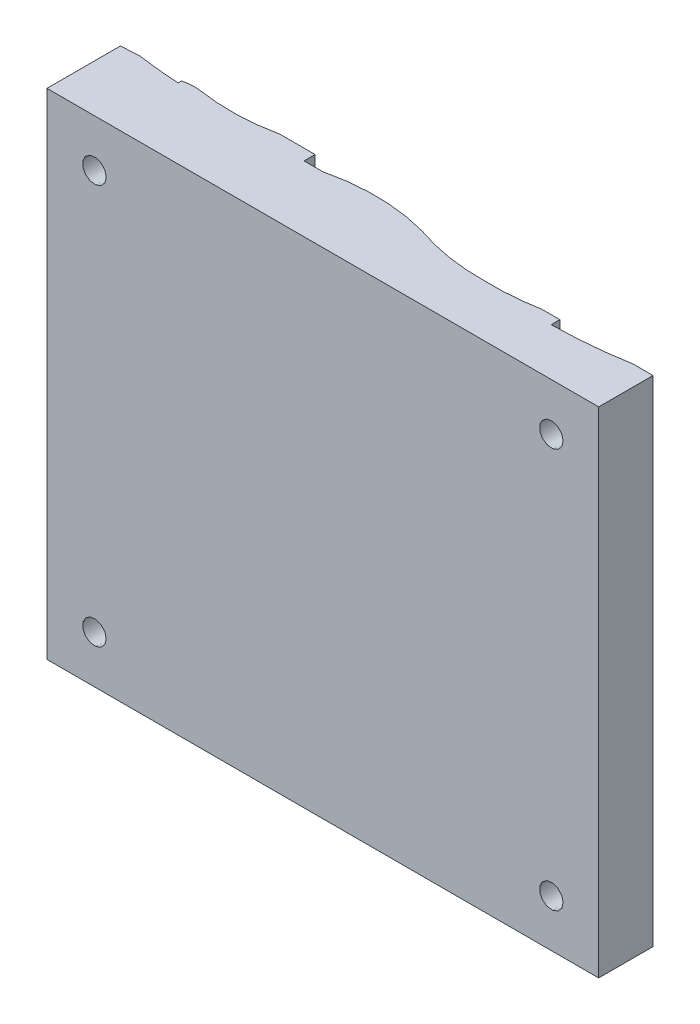
# Autodesk Inventor part: housePlate_V5
Saved by Autodesk Inventor 2023 (Build 270158000, 158)
## iProperties
Created: 2023-03-13
Part Number: housePlate_V5
Material: Generic
Document SubType Name: Modeling
Designer: shrey
Density: 1 g/cm^3
Appearance: Default
Author: shrey
Autodesk Inventor part; units mm, degrees
(part 1 of 2)
ref_plane "YZ Plane" through (0, 0, 0) normal (1, 0, 0) x (0, 1, 0)
ref_plane "XZ Plane" through (0, 0, 0) normal (0, 1, 0) x (-1, 0, 0)
ref_plane "XY Plane" through (0, 0, 0) normal (0, 0, 1) x (1, 0, 0)
ref_plane "Work Plane1" through (-64.2812, 0, 18.749) normal (0, 0, -1) x (1, 0, 0)
sketch "Sketch1" plane through (-64.2812, 0, 18.749) normal (0, 0, -1) x (1, 0, 0)
  line L0 (64.2812, -304.8) -> (64.2812, 304.8) projected
  line L1 (0, 304.8) -> (64.2812, 304.8) projected
  line L2 (0, -304.8) -> (0, 304.8) projected
  line L3 (64.2812, -304.8) -> (0, -304.8) projected
  line L4 (0, -304.8) -> (0, 304.8) projected
  line L5 (6.11, 304.8) -> (0, 304.8) projected
  line L6 (6.11, -304.8) -> (6.11, 304.8) projected
  line L7 (0, -304.8) -> (6.11, -304.8) projected
  line L8 (64.2812, 256.0593) -> (6.11, 256.0593)
  line L9 (6.11, 256.0593) -> (6.11, 203.91)
  line L10 (6.11, 203.91) -> (64.2812, 203.91)
  line L11 (64.2812, 203.91) -> (64.2812, 256.0593)
  line L12 (47.4159, 235.3375) -> (47.4159, 237.8281) construction
  arc A0 (47.4159, 237.8281) -> (43.127, 233.5392) centre (48.5159, 232.4392) ccw construction
  line L13 (43.127, 233.5392) -> (45.6176, 233.5392) construction
  arc A1 (47.4159, 235.3375) -> (45.6176, 233.5392) centre (48.5159, 232.4392) ccw construction
  circle A2 centre (48.5159, 232.4392) radius 1.1 construction
  line L14 (49.6159, 237.8281) -> (49.6159, 235.3375) construction
  arc A3 (51.4141, 233.5392) -> (49.6159, 235.3375) centre (48.5159, 232.4392) ccw construction
  line L15 (51.4141, 233.5392) -> (53.9047, 233.5392) construction
  arc A4 (53.9047, 233.5392) -> (49.6159, 237.8281) centre (48.5159, 232.4392) ccw construction
  line L16 (47.4159, 227.0503) -> (47.4159, 229.5409) construction
  arc A5 (45.6176, 231.3392) -> (47.4159, 229.5409) centre (48.5159, 232.4392) ccw construction
  line L17 (45.6176, 231.3392) -> (43.127, 231.3392) construction
  arc A6 (43.127, 231.3392) -> (47.4159, 227.0503) centre (48.5159, 232.4392) ccw construction
  line L18 (53.9047, 231.3392) -> (51.4141, 231.3392) construction
  arc A7 (49.6159, 229.5409) -> (51.4141, 231.3392) centre (48.5159, 232.4392) ccw construction
  line L19 (49.6159, 229.5409) -> (49.6159, 227.0503) construction
  arc A8 (49.6159, 227.0503) -> (53.9047, 231.3392) centre (48.5159, 232.4392) ccw construction
  spline S0 degree 3 poles (52.7785, 243.6566) (52.8138, 243.5407) (52.8843, 243.3089) (52.9667, 242.9548) (53.0306, 242.597) (53.0721, 242.2358) (53.0891, 241.8726) (53.0796, 241.5696) (53.0552, 241.3285) (53.0267, 241.1491) (52.9885, 240.9712) (52.9489, 240.8567) (52.9291, 240.7994) knots -0.290636 -0.290636 -0.290636 -0.290636 -0.254303 -0.217971 -0.18164 -0.145309 -0.10898 -0.072655 -0.054488 -0.036322 -0.018158 0 0 0 0 construction
  spline S1 degree 3 poles (52.9291, 240.7994) (52.8954, 240.7564) (52.8281, 240.6703) (52.7351, 240.5352) (52.6496, 240.3953) (52.5755, 240.249) (52.5067, 240.1001) (52.4542, 239.9447) (52.4124, 239.786) (52.3869, 239.6238) (52.3798, 239.4598) (52.3919, 239.296) (52.4259, 239.1352) (52.4842, 238.9815) (52.5637, 238.8376) (52.6499, 238.7311) (52.7267, 238.6532) (52.8128, 238.5857) (52.9249, 238.5077) (53.0338, 238.4252) (53.1246, 238.3641) (53.2224, 238.3152) (53.3503, 238.2661) (53.5117, 238.235) (53.6759, 238.227) (53.8393, 238.2444) (53.9988, 238.2835) (54.1527, 238.3409) (54.299, 238.4153) (54.437, 238.5041) (54.5686, 238.6021) (54.689, 238.7135) (54.8052, 238.8291) (54.9119, 238.9537) (55.0116, 239.0839) (55.0726, 239.1745) (55.1032, 239.2199) knots -0.524268 -0.524268 -0.524268 -0.524268 -0.507879 -0.49149 -0.475102 -0.458716 -0.44233 -0.425942 -0.409559 -0.393171 -0.376784 -0.360403 -0.344025 -0.327651 -0.311278 -0.294912 -0.286715 -0.278522 -0.262134 -0.245745 -0.237552 -0.229355 -0.21299 -0.196616 -0.180243 -0.163864 -0.147483 -0.131097 -0.114709 -0.098325 -0.081938 -0.065552 -0.049165 -0.032777 -0.016389 0 0 0 0 construction
  spline S2 degree 3 poles (55.1032, 239.2199) (55.1515, 239.2564) (55.2482, 239.3295) (55.4056, 239.4207) (55.5674, 239.5033) (55.7892, 239.601) (56.0744, 239.7036) (56.4251, 239.7997) (56.7814, 239.8718) (57.1414, 239.9217) (57.5037, 239.9527) (57.7459, 239.9573) (57.867, 239.9595) knots -0.290636 -0.290636 -0.290636 -0.290636 -0.272477 -0.254313 -0.236147 -0.217981 -0.181655 -0.145326 -0.108996 -0.072664 -0.036332 0 0 0 0 construction
  arc A9 (58.5578, 239.0087) -> (57.867, 239.9595) centre (48.5159, 232.4392) ccw construction
  spline S3 degree 3 poles (58.5578, 239.0087) (58.5182, 238.8943) (58.4391, 238.6653) (58.2976, 238.3304) (58.1389, 238.0033) (57.9602, 237.6867) (57.7605, 237.3829) (57.5747, 237.1434) (57.4133, 236.9627) (57.2848, 236.8343) (57.1493, 236.7128) (57.0499, 236.6434) (57.0003, 236.6087) knots -0.290636 -0.290636 -0.290636 -0.290636 -0.254303 -0.217971 -0.18164 -0.145309 -0.10898 -0.072655 -0.054488 -0.036322 -0.018158 0 0 0 0 construction
  spline S4 degree 3 poles (57.0003, 236.6087) (56.9477, 236.5937) (56.8427, 236.5636) (56.688, 236.509) (56.5366, 236.4461) (56.3907, 236.3713) (56.2475, 236.2913) (56.1137, 236.1963) (55.9866, 236.0926) (55.8706, 235.9764) (55.7685, 235.8478) (55.682, 235.7082) (55.6149, 235.5581) (55.5718, 235.3995) (55.5515, 235.2363) (55.5587, 235.0995) (55.575, 234.9914) (55.605, 234.8861) (55.6498, 234.7571) (55.6894, 234.6265) (55.727, 234.5237) (55.7773, 234.4266) (55.852, 234.3117) (55.9643, 234.1916) (56.0924, 234.0887) (56.2349, 234.0066) (56.3869, 233.9446) (56.5451, 233.9005) (56.7073, 233.8747) (56.871, 233.8654) (57.0351, 233.8673) (57.198, 233.8867) (57.36, 233.912) (57.5195, 233.9501) (57.6767, 233.9968) (57.7793, 234.0342) (57.8307, 234.0529) knots -0.524268 -0.524268 -0.524268 -0.524268 -0.507879 -0.49149 -0.475102 -0.458716 -0.44233 -0.425942 -0.409559 -0.393171 -0.376784 -0.360403 -0.344025 -0.327651 -0.311278 -0.294912 -0.286715 -0.278522 -0.262134 -0.245745 -0.237552 -0.229355 -0.21299 -0.196616 -0.180243 -0.163864 -0.147483 -0.131097 -0.114709 -0.098325 -0.081938 -0.065552 -0.049165 -0.032777 -0.016389 0 0 0 0 construction
  spline S5 degree 3 poles (57.8307, 234.0529) (57.8913, 234.0541) (58.0124, 234.0564) (58.1934, 234.0377) (58.3729, 234.0093) (58.6097, 233.9581) (58.9008, 233.8735) (59.2409, 233.7451) (59.5716, 233.594) (59.8922, 233.4227) (60.2035, 233.2349) (60.4022, 233.0962) (60.5015, 233.0268) knots -0.290636 -0.290636 -0.290636 -0.290636 -0.272477 -0.254313 -0.236147 -0.217981 -0.181655 -0.145326 -0.108996 -0.072664 -0.036332 0 0 0 0 construction
  arc A10 (60.5015, 231.8516) -> (60.5015, 233.0268) centre (48.5159, 232.4392) ccw construction
  spline S6 degree 3 poles (60.5015, 231.8516) (60.4022, 231.7822) (60.2035, 231.6435) (59.8922, 231.4557) (59.5716, 231.2844) (59.2409, 231.1333) (58.9008, 231.0049) (58.6097, 230.9203) (58.3729, 230.869) (58.1934, 230.8407) (58.0124, 230.822) (57.8913, 230.8243) (57.8307, 230.8254) knots -0.290636 -0.290636 -0.290636 -0.290636 -0.254303 -0.217971 -0.18164 -0.145309 -0.10898 -0.072655 -0.054488 -0.036322 -0.018158 0 0 0 0 construction
  spline S7 degree 3 poles (57.8307, 230.8254) (57.7793, 230.8441) (57.6767, 230.8815) (57.5195, 230.9283) (57.36, 230.9664) (57.198, 230.9916) (57.0351, 231.011) (56.871, 231.0129) (56.7073, 231.0036) (56.5451, 230.9778) (56.3869, 230.9338) (56.2349, 230.8717) (56.0924, 230.7897) (55.9643, 230.6868) (55.852, 230.5667) (55.7773, 230.4518) (55.727, 230.3547) (55.6894, 230.2519) (55.6498, 230.1212) (55.605, 229.9922) (55.575, 229.887) (55.5587, 229.7788) (55.5515, 229.642) (55.5718, 229.4788) (55.6149, 229.3203) (55.682, 229.1702) (55.7685, 229.0306) (55.8706, 228.902) (55.9866, 228.7858) (56.1137, 228.682) (56.2475, 228.5871) (56.3907, 228.507) (56.5366, 228.4323) (56.688, 228.3693) (56.8427, 228.3148) (56.9477, 228.2847) (57.0003, 228.2696) knots -0.524268 -0.524268 -0.524268 -0.524268 -0.507879 -0.49149 -0.475102 -0.458716 -0.44233 -0.425942 -0.409559 -0.393171 -0.376784 -0.360403 -0.344025 -0.327651 -0.311278 -0.294912 -0.286715 -0.278522 -0.262134 -0.245745 -0.237552 -0.229355 -0.21299 -0.196616 -0.180243 -0.163864 -0.147483 -0.131097 -0.114709 -0.098325 -0.081938 -0.065552 -0.049165 -0.032777 -0.016389 0 0 0 0 construction
  spline S8 degree 3 poles (57.0003, 228.2696) (57.0499, 228.235) (57.1493, 228.1656) (57.2848, 228.0441) (57.4133, 227.9157) (57.5747, 227.735) (57.7605, 227.4954) (57.9602, 227.1916) (58.1389, 226.875) (58.2976, 226.548) (58.4391, 226.2131) (58.5182, 225.9841) (58.5578, 225.8696) knots -0.290636 -0.290636 -0.290636 -0.290636 -0.272477 -0.254313 -0.236147 -0.217981 -0.181655 -0.145326 -0.108996 -0.072664 -0.036332 0 0 0 0 construction
  arc A11 (57.867, 224.9188) -> (58.5578, 225.8696) centre (48.5159, 232.4392) ccw construction
  spline S9 degree 3 poles (57.867, 224.9188) (57.7459, 224.9211) (57.5037, 224.9256) (57.1414, 224.9567) (56.7814, 225.0065) (56.4251, 225.0786) (56.0744, 225.1747) (55.7892, 225.2774) (55.5674, 225.3751) (55.4056, 225.4576) (55.2482, 225.5489) (55.1515, 225.622) (55.1032, 225.6585) knots -0.290636 -0.290636 -0.290636 -0.290636 -0.254303 -0.217971 -0.18164 -0.145309 -0.10898 -0.072655 -0.054488 -0.036322 -0.018158 0 0 0 0 construction
  spline S10 degree 3 poles (55.1032, 225.6585) (55.0726, 225.7038) (55.0116, 225.7944) (54.9119, 225.9246) (54.8052, 226.0492) (54.689, 226.1649) (54.5686, 226.2763) (54.437, 226.3743) (54.299, 226.463) (54.1527, 226.5375) (53.9988, 226.5948) (53.8393, 226.634) (53.6759, 226.6514) (53.5117, 226.6434) (53.3503, 226.6122) (53.2224, 226.5631) (53.1246, 226.5142) (53.0338, 226.4531) (52.9249, 226.3707) (52.8128, 226.2926) (52.7267, 226.2251) (52.6499, 226.1472) (52.5637, 226.0408) (52.4842, 225.8968) (52.4259, 225.7432) (52.3919, 225.5824) (52.3798, 225.4186) (52.3869, 225.2545) (52.4124, 225.0923) (52.4542, 224.9337) (52.5067, 224.7782) (52.5755, 224.6293) (52.6496, 224.4831) (52.7351, 224.3431) (52.8281, 224.2081) (52.8954, 224.122) (52.9291, 224.0789) knots -0.524268 -0.524268 -0.524268 -0.524268 -0.507879 -0.49149 -0.475102 -0.458716 -0.44233 -0.425942 -0.409559 -0.393171 -0.376784 -0.360403 -0.344025 -0.327651 -0.311278 -0.294912 -0.286715 -0.278522 -0.262134 -0.245745 -0.237552 -0.229355 -0.21299 -0.196616 -0.180243 -0.163864 -0.147483 -0.131097 -0.114709 -0.098325 -0.081938 -0.065552 -0.049165 -0.032777 -0.016389 0 0 0 0 construction
  spline S11 degree 3 poles (52.9291, 224.0789) (52.9489, 224.0217) (52.9885, 223.9072) (53.0267, 223.7293) (53.0552, 223.5498) (53.0796, 223.3087) (53.0891, 223.0058) (53.0721, 222.6426) (53.0306, 222.2814) (52.9667, 221.9235) (52.8843, 221.5694) (52.8138, 221.3377) (52.7785, 221.2218) knots -0.290636 -0.290636 -0.290636 -0.290636 -0.272477 -0.254313 -0.236147 -0.217981 -0.181655 -0.145326 -0.108996 -0.072664 -0.036332 0 0 0 0 construction
  arc A12 (51.6608, 220.8586) -> (52.7785, 221.2218) centre (48.5159, 232.4392) ccw construction
  spline S12 degree 3 poles (51.6608, 220.8586) (51.5641, 220.9316) (51.3708, 221.0777) (51.096, 221.3157) (50.834, 221.5677) (50.5881, 221.8355) (50.3609, 222.1193) (50.1905, 222.37) (50.0685, 222.5794) (49.9861, 222.7413) (49.9124, 222.9077) (49.8771, 223.0236) (49.8595, 223.0816) knots -0.290636 -0.290636 -0.290636 -0.290636 -0.254303 -0.217971 -0.18164 -0.145309 -0.10898 -0.072655 -0.054488 -0.036322 -0.018158 0 0 0 0 construction
  spline S13 degree 3 poles (49.8595, 223.0816) (49.8614, 223.1362) (49.8653, 223.2454) (49.8612, 223.4093) (49.8481, 223.5728) (49.8221, 223.7347) (49.7902, 223.8956) (49.7413, 224.0522) (49.6819, 224.2051) (49.6072, 224.3514) (49.5165, 224.4882) (49.4104, 224.6136) (49.2884, 224.7238) (49.1509, 224.8138) (49.002, 224.8835) (48.8696, 224.919) (48.7618, 224.9369) (48.6524, 224.9408) (48.5159, 224.9381) (48.3793, 224.9408) (48.27, 224.9369) (48.1621, 224.919) (48.0297, 224.8835) (47.8808, 224.8138) (47.7433, 224.7238) (47.6213, 224.6136) (47.5153, 224.4882) (47.4245, 224.3514) (47.3499, 224.2051) (47.2904, 224.0522) (47.2415, 223.8956) (47.2096, 223.7347) (47.1836, 223.5728) (47.1705, 223.4093) (47.1664, 223.2454) (47.1703, 223.1362) (47.1722, 223.0816) knots -0.524268 -0.524268 -0.524268 -0.524268 -0.507879 -0.49149 -0.475102 -0.458716 -0.44233 -0.425942 -0.409559 -0.393171 -0.376784 -0.360403 -0.344025 -0.327651 -0.311278 -0.294912 -0.286715 -0.278522 -0.262134 -0.245745 -0.237552 -0.229355 -0.21299 -0.196616 -0.180243 -0.163864 -0.147483 -0.131097 -0.114709 -0.098325 -0.081938 -0.065552 -0.049165 -0.032777 -0.016389 0 0 0 0 construction
  spline S14 degree 3 poles (47.1722, 223.0816) (47.1546, 223.0236) (47.1193, 222.9077) (47.0456, 222.7413) (46.9632, 222.5794) (46.8413, 222.37) (46.6708, 222.1193) (46.4436, 221.8355) (46.1977, 221.5677) (45.9358, 221.3157) (45.6609, 221.0777) (45.4676, 220.9316) (45.371, 220.8586) knots -0.290636 -0.290636 -0.290636 -0.290636 -0.272477 -0.254313 -0.236147 -0.217981 -0.181655 -0.145326 -0.108996 -0.072664 -0.036332 0 0 0 0 construction
  arc A13 (44.2533, 221.2218) -> (45.371, 220.8586) centre (48.5159, 232.4392) ccw construction
  spline S15 degree 3 poles (44.2533, 221.2218) (44.218, 221.3377) (44.1474, 221.5694) (44.065, 221.9235) (44.0012, 222.2814) (43.9597, 222.6426) (43.9427, 223.0058) (43.9521, 223.3087) (43.9766, 223.5498) (44.0051, 223.7293) (44.0432, 223.9072) (44.0828, 224.0217) (44.1026, 224.0789) knots -0.290636 -0.290636 -0.290636 -0.290636 -0.254303 -0.217971 -0.18164 -0.145309 -0.10898 -0.072655 -0.054488 -0.036322 -0.018158 0 0 0 0 construction
  spline S16 degree 3 poles (44.1026, 224.0789) (44.1363, 224.122) (44.2036, 224.2081) (44.2966, 224.3431) (44.3822, 224.4831) (44.4563, 224.6293) (44.525, 224.7782) (44.5775, 224.9337) (44.6193, 225.0923) (44.6449, 225.2545) (44.6519, 225.4186) (44.6398, 225.5824) (44.6059, 225.7432) (44.5475, 225.8968) (44.468, 226.0408) (44.3818, 226.1472) (44.3051, 226.2251) (44.2189, 226.2926) (44.1068, 226.3707) (43.998, 226.4531) (43.9072, 226.5142) (43.8094, 226.5631) (43.6815, 226.6122) (43.52, 226.6434) (43.3559, 226.6514) (43.1924, 226.634) (43.0329, 226.5948) (42.8791, 226.5375) (42.7327, 226.463) (42.5948, 226.3743) (42.4631, 226.2763) (42.3427, 226.1649) (42.2265, 226.0492) (42.1199, 225.9246) (42.0202, 225.7944) (41.9591, 225.7038) (41.9286, 225.6585) knots -0.524268 -0.524268 -0.524268 -0.524268 -0.507879 -0.49149 -0.475102 -0.458716 -0.44233 -0.425942 -0.409559 -0.393171 -0.376784 -0.360403 -0.344025 -0.327651 -0.311278 -0.294912 -0.286715 -0.278522 -0.262134 -0.245745 -0.237552 -0.229355 -0.21299 -0.196616 -0.180243 -0.163864 -0.147483 -0.131097 -0.114709 -0.098325 -0.081938 -0.065552 -0.049165 -0.032777 -0.016389 0 0 0 0 construction
  spline S17 degree 3 poles (41.9286, 225.6585) (41.8802, 225.622) (41.7836, 225.5489) (41.6262, 225.4576) (41.4643, 225.3751) (41.2426, 225.2774) (40.9573, 225.1747) (40.6067, 225.0786) (40.2503, 225.0065) (39.8903, 224.9567) (39.528, 224.9256) (39.2858, 224.9211) (39.1647, 224.9188) knots -0.290636 -0.290636 -0.290636 -0.290636 -0.272477 -0.254313 -0.236147 -0.217981 -0.181655 -0.145326 -0.108996 -0.072664 -0.036332 0 0 0 0 construction
  arc A14 (38.4739, 225.8696) -> (39.1647, 224.9188) centre (48.5159, 232.4392) ccw construction
  spline S18 degree 3 poles (38.4739, 225.8696) (38.5135, 225.9841) (38.5927, 226.2131) (38.7341, 226.548) (38.8928, 226.875) (39.0715, 227.1916) (39.2712, 227.4954) (39.457, 227.735) (39.6185, 227.9157) (39.747, 228.0441) (39.8824, 228.1656) (39.9818, 228.235) (40.0315, 228.2696) knots -0.290636 -0.290636 -0.290636 -0.290636 -0.254303 -0.217971 -0.18164 -0.145309 -0.10898 -0.072655 -0.054488 -0.036322 -0.018158 0 0 0 0 construction
  spline S19 degree 3 poles (40.0315, 228.2696) (40.084, 228.2847) (40.1891, 228.3148) (40.3437, 228.3693) (40.4952, 228.4323) (40.6411, 228.507) (40.7842, 228.5871) (40.9181, 228.682) (41.0451, 228.7858) (41.1611, 228.902) (41.2632, 229.0306) (41.3497, 229.1702) (41.4168, 229.3203) (41.4599, 229.4788) (41.4802, 229.642) (41.473, 229.7788) (41.4567, 229.887) (41.4267, 229.9922) (41.3819, 230.1212) (41.3423, 230.2519) (41.3048, 230.3547) (41.2544, 230.4518) (41.1798, 230.5667) (41.0674, 230.6868) (40.9394, 230.7897) (40.7969, 230.8717) (40.6448, 230.9338) (40.4867, 230.9778) (40.3245, 231.0036) (40.1607, 231.0129) (39.9966, 231.011) (39.8338, 230.9916) (39.6718, 230.9664) (39.5122, 230.9283) (39.3551, 230.8815) (39.2524, 230.8441) (39.2011, 230.8254) knots -0.524268 -0.524268 -0.524268 -0.524268 -0.507879 -0.49149 -0.475102 -0.458716 -0.44233 -0.425942 -0.409559 -0.393171 -0.376784 -0.360403 -0.344025 -0.327651 -0.311278 -0.294912 -0.286715 -0.278522 -0.262134 -0.245745 -0.237552 -0.229355 -0.21299 -0.196616 -0.180243 -0.163864 -0.147483 -0.131097 -0.114709 -0.098325 -0.081938 -0.065552 -0.049165 -0.032777 -0.016389 0 0 0 0 construction
  spline S20 degree 3 poles (39.2011, 230.8254) (39.1405, 230.8243) (39.0193, 230.822) (38.8383, 230.8407) (38.6589, 230.869) (38.422, 230.9203) (38.131, 231.0049) (37.7908, 231.1333) (37.4601, 231.2844) (37.1395, 231.4557) (36.8282, 231.6435) (36.6296, 231.7822) (36.5303, 231.8516) knots -0.290636 -0.290636 -0.290636 -0.290636 -0.272477 -0.254313 -0.236147 -0.217981 -0.181655 -0.145326 -0.108996 -0.072664 -0.036332 0 0 0 0 construction
  arc A15 (36.5303, 233.0268) -> (36.5303, 231.8516) centre (48.5159, 232.4392) ccw construction
  spline S21 degree 3 poles (36.5303, 233.0268) (36.6296, 233.0962) (36.8282, 233.2349) (37.1395, 233.4227) (37.4601, 233.594) (37.7908, 233.7451) (38.131, 233.8735) (38.422, 233.9581) (38.6589, 234.0093) (38.8383, 234.0377) (39.0193, 234.0564) (39.1405, 234.0541) (39.2011, 234.0529) knots -0.290636 -0.290636 -0.290636 -0.290636 -0.254303 -0.217971 -0.18164 -0.145309 -0.10898 -0.072655 -0.054488 -0.036322 -0.018158 0 0 0 0 construction
  spline S22 degree 3 poles (39.2011, 234.0529) (39.2524, 234.0342) (39.3551, 233.9968) (39.5122, 233.9501) (39.6718, 233.912) (39.8338, 233.8867) (39.9966, 233.8673) (40.1607, 233.8654) (40.3245, 233.8747) (40.4867, 233.9005) (40.6448, 233.9446) (40.7969, 234.0066) (40.9394, 234.0887) (41.0674, 234.1916) (41.1798, 234.3117) (41.2544, 234.4266) (41.3048, 234.5237) (41.3423, 234.6265) (41.3819, 234.7571) (41.4267, 234.8861) (41.4567, 234.9914) (41.473, 235.0995) (41.4802, 235.2363) (41.4599, 235.3995) (41.4168, 235.5581) (41.3497, 235.7082) (41.2632, 235.8478) (41.1611, 235.9764) (41.0451, 236.0926) (40.9181, 236.1963) (40.7842, 236.2913) (40.6411, 236.3713) (40.4952, 236.4461) (40.3437, 236.509) (40.1891, 236.5636) (40.084, 236.5937) (40.0315, 236.6087) knots -0.524268 -0.524268 -0.524268 -0.524268 -0.507879 -0.49149 -0.475102 -0.458716 -0.44233 -0.425942 -0.409559 -0.393171 -0.376784 -0.360403 -0.344025 -0.327651 -0.311278 -0.294912 -0.286715 -0.278522 -0.262134 -0.245745 -0.237552 -0.229355 -0.21299 -0.196616 -0.180243 -0.163864 -0.147483 -0.131097 -0.114709 -0.098325 -0.081938 -0.065552 -0.049165 -0.032777 -0.016389 0 0 0 0 construction
  spline S23 degree 3 poles (40.0315, 236.6087) (39.9818, 236.6434) (39.8824, 236.7128) (39.747, 236.8343) (39.6185, 236.9627) (39.457, 237.1434) (39.2712, 237.3829) (39.0715, 237.6867) (38.8928, 238.0033) (38.7341, 238.3304) (38.5927, 238.6653) (38.5135, 238.8943) (38.4739, 239.0087) knots -0.290636 -0.290636 -0.290636 -0.290636 -0.272477 -0.254313 -0.236147 -0.217981 -0.181655 -0.145326 -0.108996 -0.072664 -0.036332 0 0 0 0 construction
  arc A16 (39.1647, 239.9595) -> (38.4739, 239.0087) centre (48.5159, 232.4392) ccw construction
  spline S24 degree 3 poles (39.1647, 239.9595) (39.2858, 239.9573) (39.528, 239.9527) (39.8903, 239.9217) (40.2503, 239.8718) (40.6067, 239.7997) (40.9573, 239.7036) (41.2426, 239.601) (41.4643, 239.5033) (41.6262, 239.4207) (41.7836, 239.3295) (41.8802, 239.2564) (41.9286, 239.2199) knots -0.290636 -0.290636 -0.290636 -0.290636 -0.254303 -0.217971 -0.18164 -0.145309 -0.10898 -0.072655 -0.054488 -0.036322 -0.018158 0 0 0 0 construction
  spline S25 degree 3 poles (41.9286, 239.2199) (41.9591, 239.1745) (42.0202, 239.0839) (42.1199, 238.9537) (42.2265, 238.8291) (42.3427, 238.7135) (42.4631, 238.6021) (42.5948, 238.5041) (42.7327, 238.4153) (42.8791, 238.3409) (43.0329, 238.2835) (43.1924, 238.2444) (43.3559, 238.227) (43.52, 238.235) (43.6815, 238.2661) (43.8094, 238.3152) (43.9072, 238.3641) (43.998, 238.4252) (44.1068, 238.5077) (44.2189, 238.5857) (44.3051, 238.6532) (44.3818, 238.7311) (44.468, 238.8376) (44.5475, 238.9815) (44.6059, 239.1352) (44.6398, 239.296) (44.6519, 239.4598) (44.6449, 239.6238) (44.6193, 239.786) (44.5775, 239.9447) (44.525, 240.1001) (44.4563, 240.249) (44.3822, 240.3953) (44.2966, 240.5352) (44.2036, 240.6703) (44.1363, 240.7564) (44.1026, 240.7994) knots -0.524268 -0.524268 -0.524268 -0.524268 -0.507879 -0.49149 -0.475102 -0.458716 -0.44233 -0.425942 -0.409559 -0.393171 -0.376784 -0.360403 -0.344025 -0.327651 -0.311278 -0.294912 -0.286715 -0.278522 -0.262134 -0.245745 -0.237552 -0.229355 -0.21299 -0.196616 -0.180243 -0.163864 -0.147483 -0.131097 -0.114709 -0.098325 -0.081938 -0.065552 -0.049165 -0.032777 -0.016389 0 0 0 0 construction
  spline S26 degree 3 poles (44.1026, 240.7994) (44.0828, 240.8567) (44.0432, 240.9712) (44.0051, 241.1491) (43.9766, 241.3285) (43.9521, 241.5696) (43.9427, 241.8726) (43.9597, 242.2358) (44.0012, 242.597) (44.065, 242.9548) (44.1474, 243.3089) (44.218, 243.5407) (44.2533, 243.6566) knots -0.290636 -0.290636 -0.290636 -0.290636 -0.272477 -0.254313 -0.236147 -0.217981 -0.181655 -0.145326 -0.108996 -0.072664 -0.036332 0 0 0 0 construction
  arc A17 (45.371, 244.0198) -> (44.2533, 243.6566) centre (48.5159, 232.4392) ccw construction
  spline S27 degree 3 poles (45.371, 244.0198) (45.4676, 243.9467) (45.6609, 243.8007) (45.9358, 243.5626) (46.1977, 243.3107) (46.4436, 243.0429) (46.6708, 242.759) (46.8413, 242.5084) (46.9632, 242.299) (47.0456, 242.137) (47.1193, 241.9707) (47.1546, 241.8547) (47.1722, 241.7968) knots -0.290636 -0.290636 -0.290636 -0.290636 -0.254303 -0.217971 -0.18164 -0.145309 -0.10898 -0.072655 -0.054488 -0.036322 -0.018158 0 0 0 0 construction
  spline S28 degree 3 poles (47.1722, 241.7968) (47.1703, 241.7422) (47.1664, 241.633) (47.1705, 241.469) (47.1836, 241.3055) (47.2096, 241.1437) (47.2415, 240.9828) (47.2904, 240.8261) (47.3499, 240.6733) (47.4245, 240.527) (47.5153, 240.3902) (47.6213, 240.2647) (47.7433, 240.1546) (47.8808, 240.0646) (48.0297, 239.9949) (48.1621, 239.9594) (48.27, 239.9415) (48.3793, 239.9375) (48.5159, 239.9403) (48.6524, 239.9375) (48.7618, 239.9415) (48.8696, 239.9594) (49.002, 239.9949) (49.1509, 240.0646) (49.2884, 240.1546) (49.4104, 240.2647) (49.5165, 240.3902) (49.6072, 240.527) (49.6819, 240.6733) (49.7413, 240.8261) (49.7902, 240.9828) (49.8221, 241.1437) (49.8481, 241.3055) (49.8612, 241.469) (49.8653, 241.633) (49.8614, 241.7422) (49.8595, 241.7968) knots -0.524268 -0.524268 -0.524268 -0.524268 -0.507879 -0.49149 -0.475102 -0.458716 -0.44233 -0.425942 -0.409559 -0.393171 -0.376784 -0.360403 -0.344025 -0.327651 -0.311278 -0.294912 -0.286715 -0.278522 -0.262134 -0.245745 -0.237552 -0.229355 -0.21299 -0.196616 -0.180243 -0.163864 -0.147483 -0.131097 -0.114709 -0.098325 -0.081938 -0.065552 -0.049165 -0.032777 -0.016389 0 0 0 0 construction
  spline S29 degree 3 poles (49.8595, 241.7968) (49.8771, 241.8547) (49.9124, 241.9707) (49.9861, 242.137) (50.0685, 242.299) (50.1905, 242.5084) (50.3609, 242.759) (50.5881, 243.0429) (50.834, 243.3107) (51.096, 243.5626) (51.3708, 243.8007) (51.5641, 243.9467) (51.6608, 244.0198) knots -0.290636 -0.290636 -0.290636 -0.290636 -0.272477 -0.254313 -0.236147 -0.217981 -0.181655 -0.145326 -0.108996 -0.072664 -0.036332 0 0 0 0 construction
  arc A18 (52.7785, 243.6566) -> (51.6608, 244.0198) centre (48.5159, 232.4392) ccw construction
  line L20 (22.3562, 235.377) -> (22.3562, 237.8676) construction
  arc A19 (22.3562, 237.8676) -> (18.0673, 233.5787) centre (23.4562, 232.4787) ccw construction
  line L21 (18.0673, 233.5787) -> (20.5579, 233.5787) construction
  arc A20 (22.3562, 235.377) -> (20.5579, 233.5787) centre (23.4562, 232.4787) ccw construction
  circle A21 centre (23.4562, 232.4787) radius 1.1 construction
  line L22 (24.5562, 237.8676) -> (24.5562, 235.377) construction
  arc A22 (26.3545, 233.5787) -> (24.5562, 235.377) centre (23.4562, 232.4787) ccw construction
  line L23 (26.3545, 233.5787) -> (28.8451, 233.5787) construction
  arc A23 (28.8451, 233.5787) -> (24.5562, 237.8676) centre (23.4562, 232.4787) ccw construction
  line L24 (22.3562, 227.0898) -> (22.3562, 229.5804) construction
  arc A24 (20.5579, 231.3787) -> (22.3562, 229.5804) centre (23.4562, 232.4787) ccw construction
  line L25 (20.5579, 231.3787) -> (18.0673, 231.3787) construction
  arc A25 (18.0673, 231.3787) -> (22.3562, 227.0898) centre (23.4562, 232.4787) ccw construction
  line L26 (28.8451, 231.3787) -> (26.3545, 231.3787) construction
  arc A26 (24.5562, 229.5804) -> (26.3545, 231.3787) centre (23.4562, 232.4787) ccw construction
  line L27 (24.5562, 229.5804) -> (24.5562, 227.0898) construction
  arc A27 (24.5562, 227.0898) -> (28.8451, 231.3787) centre (23.4562, 232.4787) ccw construction
  spline S30 degree 3 poles (27.7188, 243.6961) (27.7541, 243.5802) (27.8246, 243.3484) (27.907, 242.9943) (27.9709, 242.6365) (28.0124, 242.2753) (28.0294, 241.9121) (28.0199, 241.6091) (27.9955, 241.3681) (27.967, 241.1886) (27.9288, 241.0107) (27.8892, 240.8962) (27.8694, 240.8389) knots -0.290636 -0.290636 -0.290636 -0.290636 -0.254303 -0.217971 -0.18164 -0.145309 -0.10898 -0.072655 -0.054488 -0.036322 -0.018158 0 0 0 0 construction
  spline S31 degree 3 poles (27.8694, 240.8389) (27.8357, 240.7959) (27.7684, 240.7098) (27.6754, 240.5748) (27.5899, 240.4348) (27.5158, 240.2886) (27.447, 240.1396) (27.3945, 239.9842) (27.3528, 239.8256) (27.3272, 239.6634) (27.3202, 239.4993) (27.3322, 239.3355) (27.3662, 239.1747) (27.4245, 239.0211) (27.504, 238.8771) (27.5902, 238.7706) (27.667, 238.6927) (27.7532, 238.6252) (27.8652, 238.5472) (27.9741, 238.4647) (28.0649, 238.4037) (28.1627, 238.3547) (28.2906, 238.3056) (28.452, 238.2745) (28.6162, 238.2665) (28.7796, 238.2839) (28.9391, 238.323) (29.093, 238.3804) (29.2394, 238.4549) (29.3773, 238.5436) (29.5089, 238.6416) (29.6293, 238.753) (29.7455, 238.8686) (29.8522, 238.9932) (29.9519, 239.1234) (30.0129, 239.2141) (30.0435, 239.2594) knots -0.524268 -0.524268 -0.524268 -0.524268 -0.507879 -0.49149 -0.475102 -0.458716 -0.44233 -0.425942 -0.409559 -0.393171 -0.376784 -0.360403 -0.344025 -0.327651 -0.311278 -0.294912 -0.286715 -0.278522 -0.262134 -0.245745 -0.237552 -0.229355 -0.21299 -0.196616 -0.180243 -0.163864 -0.147483 -0.131097 -0.114709 -0.098325 -0.081938 -0.065552 -0.049165 -0.032777 -0.016389 0 0 0 0 construction
  spline S32 degree 3 poles (30.0435, 239.2594) (30.0918, 239.2959) (30.1885, 239.369) (30.3459, 239.4602) (30.5077, 239.5428) (30.7295, 239.6405) (31.0147, 239.7432) (31.3654, 239.8392) (31.7217, 239.9114) (32.0818, 239.9612) (32.444, 239.9923) (32.6862, 239.9968) (32.8073, 239.999) knots -0.290636 -0.290636 -0.290636 -0.290636 -0.272477 -0.254313 -0.236147 -0.217981 -0.181655 -0.145326 -0.108996 -0.072664 -0.036332 0 0 0 0 construction
  arc A28 (33.4981, 239.0483) -> (32.8073, 239.999) centre (23.4562, 232.4787) ccw construction
  spline S33 degree 3 poles (33.4981, 239.0483) (33.4586, 238.9338) (33.3794, 238.7048) (33.2379, 238.3699) (33.0793, 238.0429) (32.9005, 237.7262) (32.7008, 237.4224) (32.5151, 237.1829) (32.3536, 237.0022) (32.2251, 236.8738) (32.0896, 236.7523) (31.9903, 236.6829) (31.9406, 236.6482) knots -0.290636 -0.290636 -0.290636 -0.290636 -0.254303 -0.217971 -0.18164 -0.145309 -0.10898 -0.072655 -0.054488 -0.036322 -0.018158 0 0 0 0 construction
  spline S34 degree 3 poles (31.9406, 236.6482) (31.888, 236.6332) (31.783, 236.6031) (31.6284, 236.5486) (31.4769, 236.4856) (31.331, 236.4108) (31.1878, 236.3308) (31.054, 236.2359) (30.927, 236.1321) (30.8109, 236.0159) (30.7088, 235.8873) (30.6223, 235.7477) (30.5552, 235.5976) (30.5121, 235.439) (30.4918, 235.2759) (30.499, 235.139) (30.5153, 235.0309) (30.5454, 234.9257) (30.5901, 234.7967) (30.6297, 234.666) (30.6673, 234.5632) (30.7177, 234.4661) (30.7923, 234.3512) (30.9046, 234.2311) (31.0327, 234.1282) (31.1752, 234.0462) (31.3272, 233.9841) (31.4854, 233.94) (31.6476, 233.9143) (31.8113, 233.905) (31.9754, 233.9069) (32.1383, 233.9262) (32.3003, 233.9515) (32.4598, 233.9896) (32.617, 234.0363) (32.7197, 234.0738) (32.771, 234.0925) knots -0.524268 -0.524268 -0.524268 -0.524268 -0.507879 -0.49149 -0.475102 -0.458716 -0.44233 -0.425942 -0.409559 -0.393171 -0.376784 -0.360403 -0.344025 -0.327651 -0.311278 -0.294912 -0.286715 -0.278522 -0.262134 -0.245745 -0.237552 -0.229355 -0.21299 -0.196616 -0.180243 -0.163864 -0.147483 -0.131097 -0.114709 -0.098325 -0.081938 -0.065552 -0.049165 -0.032777 -0.016389 0 0 0 0 construction
  spline S35 degree 3 poles (32.771, 234.0925) (32.8316, 234.0936) (32.9527, 234.0959) (33.1337, 234.0772) (33.3132, 234.0489) (33.55, 233.9976) (33.8411, 233.913) (34.1813, 233.7846) (34.5119, 233.6335) (34.8325, 233.4622) (35.1438, 233.2744) (35.3425, 233.1357) (35.4418, 233.0663) knots -0.290636 -0.290636 -0.290636 -0.290636 -0.272477 -0.254313 -0.236147 -0.217981 -0.181655 -0.145326 -0.108996 -0.072664 -0.036332 0 0 0 0 construction
  arc A29 (35.4418, 231.8911) -> (35.4418, 233.0663) centre (23.4562, 232.4787) ccw construction
  spline S36 degree 3 poles (35.4418, 231.8911) (35.3425, 231.8217) (35.1438, 231.683) (34.8325, 231.4952) (34.5119, 231.3239) (34.1813, 231.1728) (33.8411, 231.0444) (33.55, 230.9598) (33.3132, 230.9085) (33.1337, 230.8802) (32.9527, 230.8615) (32.8316, 230.8638) (32.771, 230.8649) knots -0.290636 -0.290636 -0.290636 -0.290636 -0.254303 -0.217971 -0.18164 -0.145309 -0.10898 -0.072655 -0.054488 -0.036322 -0.018158 0 0 0 0 construction
  spline S37 degree 3 poles (32.771, 230.8649) (32.7197, 230.8836) (32.617, 230.921) (32.4598, 230.9678) (32.3003, 231.0059) (32.1383, 231.0312) (31.9754, 231.0505) (31.8113, 231.0524) (31.6476, 231.0431) (31.4854, 231.0174) (31.3272, 230.9733) (31.1752, 230.9112) (31.0327, 230.8292) (30.9046, 230.7263) (30.7923, 230.6062) (30.7177, 230.4913) (30.6673, 230.3942) (30.6297, 230.2914) (30.5901, 230.1607) (30.5454, 230.0317) (30.5153, 229.9265) (30.499, 229.8184) (30.4918, 229.6815) (30.5121, 229.5183) (30.5552, 229.3598) (30.6223, 229.2097) (30.7088, 229.0701) (30.8109, 228.9415) (30.927, 228.8253) (31.054, 228.7215) (31.1878, 228.6266) (31.331, 228.5466) (31.4769, 228.4718) (31.6284, 228.4088) (31.783, 228.3543) (31.888, 228.3242) (31.9406, 228.3091) knots -0.524268 -0.524268 -0.524268 -0.524268 -0.507879 -0.49149 -0.475102 -0.458716 -0.44233 -0.425942 -0.409559 -0.393171 -0.376784 -0.360403 -0.344025 -0.327651 -0.311278 -0.294912 -0.286715 -0.278522 -0.262134 -0.245745 -0.237552 -0.229355 -0.21299 -0.196616 -0.180243 -0.163864 -0.147483 -0.131097 -0.114709 -0.098325 -0.081938 -0.065552 -0.049165 -0.032777 -0.016389 0 0 0 0 construction
  spline S38 degree 3 poles (31.9406, 228.3091) (31.9903, 228.2745) (32.0896, 228.2051) (32.2251, 228.0836) (32.3536, 227.9552) (32.5151, 227.7745) (32.7008, 227.535) (32.9005, 227.2311) (33.0793, 226.9145) (33.2379, 226.5875) (33.3794, 226.2526) (33.4586, 226.0236) (33.4981, 225.9091) knots -0.290636 -0.290636 -0.290636 -0.290636 -0.272477 -0.254313 -0.236147 -0.217981 -0.181655 -0.145326 -0.108996 -0.072664 -0.036332 0 0 0 0 construction
  arc A30 (32.8073, 224.9583) -> (33.4981, 225.9091) centre (23.4562, 232.4787) ccw construction
  spline S39 degree 3 poles (32.8073, 224.9583) (32.6862, 224.9606) (32.444, 224.9651) (32.0818, 224.9962) (31.7217, 225.046) (31.3654, 225.1182) (31.0147, 225.2142) (30.7295, 225.3169) (30.5077, 225.4146) (30.3459, 225.4972) (30.1885, 225.5884) (30.0918, 225.6615) (30.0435, 225.698) knots -0.290636 -0.290636 -0.290636 -0.290636 -0.254303 -0.217971 -0.18164 -0.145309 -0.10898 -0.072655 -0.054488 -0.036322 -0.018158 0 0 0 0 construction
  spline S40 degree 3 poles (30.0435, 225.698) (30.0129, 225.7433) (29.9519, 225.8339) (29.8522, 225.9641) (29.7455, 226.0887) (29.6293, 226.2044) (29.5089, 226.3158) (29.3773, 226.4138) (29.2394, 226.5025) (29.093, 226.577) (28.9391, 226.6343) (28.7796, 226.6735) (28.6162, 226.6909) (28.452, 226.6829) (28.2906, 226.6518) (28.1627, 226.6027) (28.0649, 226.5537) (27.9741, 226.4926) (27.8652, 226.4102) (27.7532, 226.3321) (27.667, 226.2647) (27.5902, 226.1868) (27.504, 226.0803) (27.4245, 225.9363) (27.3662, 225.7827) (27.3322, 225.6219) (27.3202, 225.4581) (27.3272, 225.294) (27.3528, 225.1318) (27.3945, 224.9732) (27.447, 224.8177) (27.5158, 224.6688) (27.5899, 224.5226) (27.6754, 224.3826) (27.7684, 224.2476) (27.8357, 224.1615) (27.8694, 224.1185) knots -0.524268 -0.524268 -0.524268 -0.524268 -0.507879 -0.49149 -0.475102 -0.458716 -0.44233 -0.425942 -0.409559 -0.393171 -0.376784 -0.360403 -0.344025 -0.327651 -0.311278 -0.294912 -0.286715 -0.278522 -0.262134 -0.245745 -0.237552 -0.229355 -0.21299 -0.196616 -0.180243 -0.163864 -0.147483 -0.131097 -0.114709 -0.098325 -0.081938 -0.065552 -0.049165 -0.032777 -0.016389 0 0 0 0 construction
  spline S41 degree 3 poles (27.8694, 224.1185) (27.8892, 224.0612) (27.9288, 223.9467) (27.967, 223.7688) (27.9955, 223.5893) (28.0199, 223.3483) (28.0294, 223.0453) (28.0124, 222.6821) (27.9709, 222.3209) (27.907, 221.9631) (27.8246, 221.6089) (27.7541, 221.3772) (27.7188, 221.2613) knots -0.290636 -0.290636 -0.290636 -0.290636 -0.272477 -0.254313 -0.236147 -0.217981 -0.181655 -0.145326 -0.108996 -0.072664 -0.036332 0 0 0 0 construction
  arc A31 (26.6011, 220.8981) -> (27.7188, 221.2613) centre (23.4562, 232.4787) ccw construction
  spline S42 degree 3 poles (26.6011, 220.8981) (26.5044, 220.9711) (26.3111, 221.1172) (26.0363, 221.3552) (25.7743, 221.6072) (25.5284, 221.875) (25.3012, 222.1588) (25.1308, 222.4095) (25.0089, 222.6189) (24.9264, 222.7808) (24.8527, 222.9472) (24.8175, 223.0631) (24.7998, 223.1211) knots -0.290636 -0.290636 -0.290636 -0.290636 -0.254303 -0.217971 -0.18164 -0.145309 -0.10898 -0.072655 -0.054488 -0.036322 -0.018158 0 0 0 0 construction
  spline S43 degree 3 poles (24.7998, 223.1211) (24.8018, 223.1757) (24.8056, 223.2849) (24.8015, 223.4488) (24.7884, 223.6123) (24.7624, 223.7742) (24.7305, 223.9351) (24.6816, 224.0917) (24.6222, 224.2446) (24.5475, 224.3909) (24.4568, 224.5277) (24.3507, 224.6531) (24.2287, 224.7633) (24.0912, 224.8533) (23.9423, 224.923) (23.81, 224.9585) (23.7021, 224.9764) (23.5927, 224.9803) (23.4562, 224.9776) (23.3197, 224.9803) (23.2103, 224.9764) (23.1024, 224.9585) (22.9701, 224.923) (22.8211, 224.8533) (22.6837, 224.7633) (22.5616, 224.6531) (22.4556, 224.5277) (22.3648, 224.3909) (22.2902, 224.2446) (22.2308, 224.0917) (22.1819, 223.9351) (22.1499, 223.7742) (22.1239, 223.6123) (22.1109, 223.4488) (22.1067, 223.2849) (22.1106, 223.1757) (22.1125, 223.1211) knots -0.524268 -0.524268 -0.524268 -0.524268 -0.507879 -0.49149 -0.475102 -0.458716 -0.44233 -0.425942 -0.409559 -0.393171 -0.376784 -0.360403 -0.344025 -0.327651 -0.311278 -0.294912 -0.286715 -0.278522 -0.262134 -0.245745 -0.237552 -0.229355 -0.21299 -0.196616 -0.180243 -0.163864 -0.147483 -0.131097 -0.114709 -0.098325 -0.081938 -0.065552 -0.049165 -0.032777 -0.016389 0 0 0 0 construction
  spline S44 degree 3 poles (22.1125, 223.1211) (22.0949, 223.0631) (22.0596, 222.9472) (21.9859, 222.7808) (21.9035, 222.6189) (21.7816, 222.4095) (21.6112, 222.1588) (21.3839, 221.875) (21.138, 221.6072) (20.8761, 221.3552) (20.6012, 221.1172) (20.4079, 220.9711) (20.3113, 220.8981) knots -0.290636 -0.290636 -0.290636 -0.290636 -0.272477 -0.254313 -0.236147 -0.217981 -0.181655 -0.145326 -0.108996 -0.072664 -0.036332 0 0 0 0 construction
  arc A32 (19.1936, 221.2613) -> (20.3113, 220.8981) centre (23.4562, 232.4787) ccw construction
  spline S45 degree 3 poles (19.1936, 221.2613) (19.1583, 221.3772) (19.0877, 221.6089) (19.0053, 221.9631) (18.9415, 222.3209) (18.9, 222.6821) (18.883, 223.0453) (18.8925, 223.3483) (18.9169, 223.5893) (18.9454, 223.7688) (18.9835, 223.9467) (19.0232, 224.0612) (19.043, 224.1185) knots -0.290636 -0.290636 -0.290636 -0.290636 -0.254303 -0.217971 -0.18164 -0.145309 -0.10898 -0.072655 -0.054488 -0.036322 -0.018158 0 0 0 0 construction
  spline S46 degree 3 poles (19.043, 224.1185) (19.0766, 224.1615) (19.1439, 224.2476) (19.237, 224.3826) (19.3225, 224.5226) (19.3966, 224.6688) (19.4653, 224.8177) (19.5178, 224.9732) (19.5596, 225.1318) (19.5852, 225.294) (19.5922, 225.4581) (19.5801, 225.6219) (19.5462, 225.7827) (19.4878, 225.9363) (19.4083, 226.0803) (19.3221, 226.1868) (19.2454, 226.2647) (19.1592, 226.3321) (19.0472, 226.4102) (18.9383, 226.4926) (18.8475, 226.5537) (18.7497, 226.6027) (18.6218, 226.6518) (18.4603, 226.6829) (18.2962, 226.6909) (18.1327, 226.6735) (17.9732, 226.6343) (17.8194, 226.577) (17.673, 226.5025) (17.5351, 226.4138) (17.4034, 226.3158) (17.283, 226.2044) (17.1669, 226.0887) (17.0602, 225.9641) (16.9605, 225.8339) (16.8994, 225.7433) (16.8689, 225.698) knots -0.524268 -0.524268 -0.524268 -0.524268 -0.507879 -0.49149 -0.475102 -0.458716 -0.44233 -0.425942 -0.409559 -0.393171 -0.376784 -0.360403 -0.344025 -0.327651 -0.311278 -0.294912 -0.286715 -0.278522 -0.262134 -0.245745 -0.237552 -0.229355 -0.21299 -0.196616 -0.180243 -0.163864 -0.147483 -0.131097 -0.114709 -0.098325 -0.081938 -0.065552 -0.049165 -0.032777 -0.016389 0 0 0 0 construction
  spline S47 degree 3 poles (16.8689, 225.698) (16.8206, 225.6615) (16.7239, 225.5884) (16.5665, 225.4972) (16.4046, 225.4146) (16.1829, 225.3169) (15.8977, 225.2142) (15.547, 225.1182) (15.1907, 225.046) (14.8306, 224.9962) (14.4684, 224.9651) (14.2261, 224.9606) (14.105, 224.9583) knots -0.290636 -0.290636 -0.290636 -0.290636 -0.272477 -0.254313 -0.236147 -0.217981 -0.181655 -0.145326 -0.108996 -0.072664 -0.036332 0 0 0 0 construction
  arc A33 (13.4142, 225.9091) -> (14.105, 224.9583) centre (23.4562, 232.4787) ccw construction
  spline S48 degree 3 poles (13.4142, 225.9091) (13.4538, 226.0236) (13.533, 226.2526) (13.6744, 226.5875) (13.8331, 226.9145) (14.0118, 227.2311) (14.2116, 227.535) (14.3973, 227.7745) (14.5588, 227.9552) (14.6873, 228.0836) (14.8227, 228.2051) (14.9221, 228.2745) (14.9718, 228.3091) knots -0.290636 -0.290636 -0.290636 -0.290636 -0.254303 -0.217971 -0.18164 -0.145309 -0.10898 -0.072655 -0.054488 -0.036322 -0.018158 0 0 0 0 construction
  spline S49 degree 3 poles (14.9718, 228.3091) (15.0243, 228.3242) (15.1294, 228.3543) (15.284, 228.4088) (15.4355, 228.4718) (15.5814, 228.5466) (15.7245, 228.6266) (15.8584, 228.7215) (15.9854, 228.8253) (16.1015, 228.9415) (16.2036, 229.0701) (16.2901, 229.2097) (16.3571, 229.3598) (16.4002, 229.5183) (16.4205, 229.6815) (16.4133, 229.8184) (16.397, 229.9265) (16.367, 230.0317) (16.3222, 230.1607) (16.2826, 230.2914) (16.2451, 230.3942) (16.1947, 230.4913) (16.1201, 230.6062) (16.0077, 230.7263) (15.8797, 230.8292) (15.7372, 230.9112) (15.5852, 230.9733) (15.427, 231.0174) (15.2648, 231.0431) (15.101, 231.0524) (14.937, 231.0505) (14.7741, 231.0312) (14.6121, 231.0059) (14.4525, 230.9678) (14.2954, 230.921) (14.1927, 230.8836) (14.1414, 230.8649) knots -0.524268 -0.524268 -0.524268 -0.524268 -0.507879 -0.49149 -0.475102 -0.458716 -0.44233 -0.425942 -0.409559 -0.393171 -0.376784 -0.360403 -0.344025 -0.327651 -0.311278 -0.294912 -0.286715 -0.278522 -0.262134 -0.245745 -0.237552 -0.229355 -0.21299 -0.196616 -0.180243 -0.163864 -0.147483 -0.131097 -0.114709 -0.098325 -0.081938 -0.065552 -0.049165 -0.032777 -0.016389 0 0 0 0 construction
  spline S50 degree 3 poles (14.1414, 230.8649) (14.0808, 230.8638) (13.9596, 230.8615) (13.7786, 230.8802) (13.5992, 230.9085) (13.3623, 230.9598) (13.0713, 231.0444) (12.7311, 231.1728) (12.4004, 231.3239) (12.0798, 231.4952) (11.7685, 231.683) (11.5699, 231.8217) (11.4706, 231.8911) knots -0.290636 -0.290636 -0.290636 -0.290636 -0.272477 -0.254313 -0.236147 -0.217981 -0.181655 -0.145326 -0.108996 -0.072664 -0.036332 0 0 0 0 construction
  arc A34 (11.4706, 233.0663) -> (11.4706, 231.8911) centre (23.4562, 232.4787) ccw construction
  spline S51 degree 3 poles (11.4706, 233.0663) (11.5699, 233.1357) (11.7685, 233.2744) (12.0798, 233.4622) (12.4004, 233.6335) (12.7311, 233.7846) (13.0713, 233.913) (13.3623, 233.9976) (13.5992, 234.0489) (13.7786, 234.0772) (13.9596, 234.0959) (14.0808, 234.0936) (14.1414, 234.0925) knots -0.290636 -0.290636 -0.290636 -0.290636 -0.254303 -0.217971 -0.18164 -0.145309 -0.10898 -0.072655 -0.054488 -0.036322 -0.018158 0 0 0 0 construction
  spline S52 degree 3 poles (14.1414, 234.0925) (14.1927, 234.0738) (14.2954, 234.0363) (14.4525, 233.9896) (14.6121, 233.9515) (14.7741, 233.9262) (14.937, 233.9069) (15.101, 233.905) (15.2648, 233.9143) (15.427, 233.94) (15.5852, 233.9841) (15.7372, 234.0462) (15.8797, 234.1282) (16.0077, 234.2311) (16.1201, 234.3512) (16.1947, 234.4661) (16.2451, 234.5632) (16.2826, 234.666) (16.3222, 234.7967) (16.367, 234.9257) (16.397, 235.0309) (16.4133, 235.139) (16.4205, 235.2759) (16.4002, 235.439) (16.3571, 235.5976) (16.2901, 235.7477) (16.2036, 235.8873) (16.1015, 236.0159) (15.9854, 236.1321) (15.8584, 236.2359) (15.7245, 236.3308) (15.5814, 236.4108) (15.4355, 236.4856) (15.284, 236.5486) (15.1294, 236.6031) (15.0243, 236.6332) (14.9718, 236.6482) knots -0.524268 -0.524268 -0.524268 -0.524268 -0.507879 -0.49149 -0.475102 -0.458716 -0.44233 -0.425942 -0.409559 -0.393171 -0.376784 -0.360403 -0.344025 -0.327651 -0.311278 -0.294912 -0.286715 -0.278522 -0.262134 -0.245745 -0.237552 -0.229355 -0.21299 -0.196616 -0.180243 -0.163864 -0.147483 -0.131097 -0.114709 -0.098325 -0.081938 -0.065552 -0.049165 -0.032777 -0.016389 0 0 0 0 construction
  spline S53 degree 3 poles (14.9718, 236.6482) (14.9221, 236.6829) (14.8227, 236.7523) (14.6873, 236.8738) (14.5588, 237.0022) (14.3973, 237.1829) (14.2116, 237.4224) (14.0118, 237.7262) (13.8331, 238.0429) (13.6744, 238.3699) (13.533, 238.7048) (13.4538, 238.9338) (13.4142, 239.0483) knots -0.290636 -0.290636 -0.290636 -0.290636 -0.272477 -0.254313 -0.236147 -0.217981 -0.181655 -0.145326 -0.108996 -0.072664 -0.036332 0 0 0 0 construction
  arc A35 (14.105, 239.999) -> (13.4142, 239.0483) centre (23.4562, 232.4787) ccw construction
  spline S54 degree 3 poles (14.105, 239.999) (14.2261, 239.9968) (14.4684, 239.9923) (14.8306, 239.9612) (15.1907, 239.9114) (15.547, 239.8392) (15.8977, 239.7432) (16.1829, 239.6405) (16.4046, 239.5428) (16.5665, 239.4602) (16.7239, 239.369) (16.8206, 239.2959) (16.8689, 239.2594) knots -0.290636 -0.290636 -0.290636 -0.290636 -0.254303 -0.217971 -0.18164 -0.145309 -0.10898 -0.072655 -0.054488 -0.036322 -0.018158 0 0 0 0 construction
  spline S55 degree 3 poles (16.8689, 239.2594) (16.8994, 239.2141) (16.9605, 239.1234) (17.0602, 238.9932) (17.1669, 238.8686) (17.283, 238.753) (17.4034, 238.6416) (17.5351, 238.5436) (17.673, 238.4549) (17.8194, 238.3804) (17.9732, 238.323) (18.1327, 238.2839) (18.2962, 238.2665) (18.4603, 238.2745) (18.6218, 238.3056) (18.7497, 238.3547) (18.8475, 238.4037) (18.9383, 238.4647) (19.0472, 238.5472) (19.1592, 238.6252) (19.2454, 238.6927) (19.3221, 238.7706) (19.4083, 238.8771) (19.4878, 239.0211) (19.5462, 239.1747) (19.5801, 239.3355) (19.5922, 239.4993) (19.5852, 239.6634) (19.5596, 239.8256) (19.5178, 239.9842) (19.4653, 240.1396) (19.3966, 240.2886) (19.3225, 240.4348) (19.237, 240.5748) (19.1439, 240.7098) (19.0766, 240.7959) (19.043, 240.8389) knots -0.524268 -0.524268 -0.524268 -0.524268 -0.507879 -0.49149 -0.475102 -0.458716 -0.44233 -0.425942 -0.409559 -0.393171 -0.376784 -0.360403 -0.344025 -0.327651 -0.311278 -0.294912 -0.286715 -0.278522 -0.262134 -0.245745 -0.237552 -0.229355 -0.21299 -0.196616 -0.180243 -0.163864 -0.147483 -0.131097 -0.114709 -0.098325 -0.081938 -0.065552 -0.049165 -0.032777 -0.016389 0 0 0 0 construction
  spline S56 degree 3 poles (19.043, 240.8389) (19.0232, 240.8962) (18.9835, 241.0107) (18.9454, 241.1886) (18.9169, 241.3681) (18.8925, 241.6091) (18.883, 241.9121) (18.9, 242.2753) (18.9415, 242.6365) (19.0053, 242.9943) (19.0877, 243.3484) (19.1583, 243.5802) (19.1936, 243.6961) knots -0.290636 -0.290636 -0.290636 -0.290636 -0.272477 -0.254313 -0.236147 -0.217981 -0.181655 -0.145326 -0.108996 -0.072664 -0.036332 0 0 0 0 construction
  arc A36 (20.3113, 244.0593) -> (19.1936, 243.6961) centre (23.4562, 232.4787) ccw construction
  spline S57 degree 3 poles (20.3113, 244.0593) (20.4079, 243.9862) (20.6012, 243.8402) (20.8761, 243.6022) (21.138, 243.3502) (21.3839, 243.0824) (21.6112, 242.7986) (21.7816, 242.5479) (21.9035, 242.3385) (21.9859, 242.1766) (22.0596, 242.0102) (22.0949, 241.8943) (22.1125, 241.8363) knots -0.290636 -0.290636 -0.290636 -0.290636 -0.254303 -0.217971 -0.18164 -0.145309 -0.10898 -0.072655 -0.054488 -0.036322 -0.018158 0 0 0 0 construction
  spline S58 degree 3 poles (22.1125, 241.8363) (22.1106, 241.7817) (22.1067, 241.6725) (22.1109, 241.5086) (22.1239, 241.345) (22.1499, 241.1832) (22.1819, 241.0223) (22.2308, 240.8656) (22.2902, 240.7128) (22.3648, 240.5665) (22.4556, 240.4297) (22.5616, 240.3043) (22.6837, 240.1941) (22.8211, 240.1041) (22.9701, 240.0344) (23.1024, 239.9989) (23.2103, 239.981) (23.3197, 239.9771) (23.4562, 239.9798) (23.5927, 239.9771) (23.7021, 239.981) (23.81, 239.9989) (23.9423, 240.0344) (24.0912, 240.1041) (24.2287, 240.1941) (24.3507, 240.3043) (24.4568, 240.4297) (24.5475, 240.5665) (24.6222, 240.7128) (24.6816, 240.8656) (24.7305, 241.0223) (24.7624, 241.1832) (24.7884, 241.345) (24.8015, 241.5086) (24.8056, 241.6725) (24.8018, 241.7817) (24.7998, 241.8363) knots -0.524268 -0.524268 -0.524268 -0.524268 -0.507879 -0.49149 -0.475102 -0.458716 -0.44233 -0.425942 -0.409559 -0.393171 -0.376784 -0.360403 -0.344025 -0.327651 -0.311278 -0.294912 -0.286715 -0.278522 -0.262134 -0.245745 -0.237552 -0.229355 -0.21299 -0.196616 -0.180243 -0.163864 -0.147483 -0.131097 -0.114709 -0.098325 -0.081938 -0.065552 -0.049165 -0.032777 -0.016389 0 0 0 0 construction
  spline S59 degree 3 poles (24.7998, 241.8363) (24.8175, 241.8943) (24.8527, 242.0102) (24.9264, 242.1766) (25.0089, 242.3385) (25.1308, 242.5479) (25.3012, 242.7986) (25.5284, 243.0824) (25.7743, 243.3502) (26.0363, 243.6022) (26.3111, 243.8402) (26.5044, 243.9862) (26.6011, 244.0593) knots -0.290636 -0.290636 -0.290636 -0.290636 -0.272477 -0.254313 -0.236147 -0.217981 -0.181655 -0.145326 -0.108996 -0.072664 -0.036332 0 0 0 0 construction
  arc A37 (27.7188, 243.6961) -> (26.6011, 244.0593) centre (23.4562, 232.4787) ccw construction
  spline S60 degree 3 poles (-19.9828, 223.4534) (-19.863, 223.2633) (-19.6832, 222.9781) (-19.4622, 222.5867) (-19.3034, 222.2894) (-19.1529, 221.9878) (-19.0111, 221.6819) (-18.8791, 221.3718) (-18.7577, 221.0573) (-18.6487, 220.7383) (-18.5527, 220.415) (-18.4903, 220.1411) (-18.4452, 219.921) (-18.3975, 219.7591) (-18.3331, 219.6031) (-18.2492, 219.4564) (-18.1607, 219.3467) (-18.0808, 219.2675) (-18.0132, 219.217) (-17.944, 219.1686) (-17.8677, 219.1325) (-17.7902, 219.099) (-17.7081, 219.0792) (-17.6254, 219.0625) (-17.5128, 219.0585) (-17.3725, 219.061) (-17.2321, 219.0585) (-17.1195, 219.0625) (-17.0368, 219.0792) (-16.9547, 219.099) (-16.8772, 219.1325) (-16.8009, 219.1686) (-16.7317, 219.217) (-16.6641, 219.2675) (-16.5842, 219.3467) (-16.4958, 219.4564) (-16.4118, 219.6031) (-16.3474, 219.7591) (-16.2998, 219.921) (-16.2547, 220.1411) (-16.1922, 220.415) (-16.0963, 220.7383) (-15.9872, 221.0573) (-15.8658, 221.3718) (-15.7338, 221.6819) (-15.5921, 221.9878) (-15.4416, 222.2894) (-15.2827, 222.5867) (-15.0617, 222.9781) (-14.8819, 223.2633) (-14.7621, 223.4534) knots -1.0784 -1.0784 -1.0784 -1.0784 -1.010995 -0.977291 -0.943586 -0.909882 -0.876178 -0.842474 -0.80877 -0.775067 -0.741365 -0.707665 -0.690816 -0.67397 -0.657123 -0.640284 -0.623449 -0.615023 -0.606598 -0.598176 -0.589749 -0.581327 -0.572901 -0.564477 -0.556053 -0.5392 -0.522347 -0.513923 -0.505499 -0.497074 -0.488651 -0.480225 -0.471802 -0.463377 -0.454951 -0.438116 -0.421277 -0.40443 -0.387584 -0.370735 -0.337035 -0.303333 -0.26963 -0.235926 -0.202222 -0.168518 -0.134814 -0.101109 -0.067405 0 0 0 0 construction
  line L28 (-14.7621, 223.4534) -> (-13.6998, 223.4534) construction
  spline S61 degree 3 poles (-13.6998, 223.4534) (-13.58, 223.2633) (-13.4002, 222.9781) (-13.1792, 222.5867) (-13.0204, 222.2894) (-12.8699, 221.9878) (-12.7281, 221.6819) (-12.5961, 221.3718) (-12.4747, 221.0573) (-12.3657, 220.7383) (-12.2697, 220.415) (-12.2073, 220.1411) (-12.1622, 219.921) (-12.1145, 219.7591) (-12.0501, 219.6031) (-11.9662, 219.4564) (-11.8777, 219.3467) (-11.7978, 219.2675) (-11.7302, 219.217) (-11.661, 219.1686) (-11.5847, 219.1325) (-11.5072, 219.099) (-11.4251, 219.0792) (-11.3424, 219.0625) (-11.2298, 219.0585) (-11.0895, 219.061) (-10.9491, 219.0585) (-10.8365, 219.0625) (-10.7538, 219.0792) (-10.6717, 219.099) (-10.5942, 219.1325) (-10.5179, 219.1686) (-10.4487, 219.217) (-10.3811, 219.2675) (-10.3012, 219.3467) (-10.2128, 219.4564) (-10.1288, 219.6031) (-10.0644, 219.7591) (-10.0168, 219.921) (-9.9717, 220.1411) (-9.9092, 220.415) (-9.8133, 220.7383) (-9.7042, 221.0573) (-9.5828, 221.3718) (-9.4508, 221.6819) (-9.3091, 221.9878) (-9.1586, 222.2894) (-8.9997, 222.5867) (-8.7787, 222.9781) (-8.5989, 223.2633) (-8.4791, 223.4534) knots -1.0784 -1.0784 -1.0784 -1.0784 -1.010995 -0.977291 -0.943586 -0.909882 -0.876178 -0.842474 -0.80877 -0.775067 -0.741365 -0.707665 -0.690816 -0.67397 -0.657123 -0.640284 -0.623449 -0.615023 -0.606598 -0.598176 -0.589749 -0.581327 -0.572901 -0.564477 -0.556053 -0.5392 -0.522347 -0.513923 -0.505499 -0.497074 -0.488651 -0.480225 -0.471802 -0.463377 -0.454951 -0.438116 -0.421277 -0.40443 -0.387584 -0.370735 -0.337035 -0.303333 -0.26963 -0.235926 -0.202222 -0.168518 -0.134814 -0.101109 -0.067405 0 0 0 0 construction
  line L29 (-8.4791, 223.4534) -> (-7.4168, 223.4534) construction